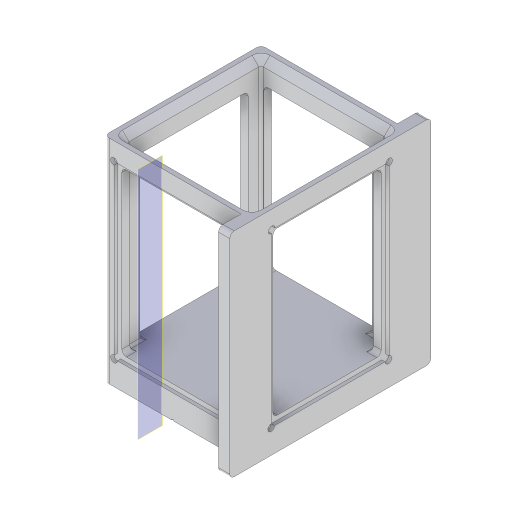
# Autodesk Inventor part: cuvette-w70mm-slide50x75mm-v1
Saved by Autodesk Inventor 2024 (Build 280153000, 153)
## iProperties
Created: 2025-09-30
Part Number: cuvette-w70mm-slide50x75mm-v1
Material: Generic
Document SubType Name: Modeling
Designer: N.Vladimirov
Density: 1 g/cm^3
Appearance: Default
Author: N.Vladimirov
Autodesk Inventor part; units mm, degrees
ref_plane "YZ Plane" through (0, 0, 0) normal (1, 0, 0) x (0, 1, 0)
ref_plane "XZ Plane" through (0, 0, 0) normal (0, 1, 0) x (-1, 0, 0)
ref_plane "XY Plane" through (0, 0, 0) normal (0, 0, 1) x (1, 0, 0)
sketch "Sketch1" plane through (0, 0, 0) normal (0, 0, 1) x (1, 0, 0)
  line L0 (30.5, -35) -> (-30.5, -35)
  line L1 (-30.5, -35) -> (-30.5, 35)
  line L2 (-30.5, 35) -> (30.5, 35)
  line L3 (30.5, 35) -> (30.5, -35)
  line L4 (30.5, -35) -> (-30.5, 35) construction
  line L5 (-30.5, -35) -> (30.5, 35) construction
  point P0 (0, 0)
  dimension "d0" = 61
  dimension "d1" = 70
  constraints: 12 end point, 2 midpoint, 2 parallel, 1 horizontal, 1 perpendicular
  measures "d0" distance of L1.end L2.end
  measures "d1" distance of L0.end L1.end
sketch "Sketch1 outline for Extrusion1" plane through (0, 0, 0) normal (0, 0, 1) x (1, 0, 0)
  line L0 (30.5, -35) -> (30.5, 35)
  line L1 (-30.5, -35) -> (30.5, -35)
  line L2 (-30.5, 35) -> (-30.5, -35)
  line L3 (30.5, 35) -> (-30.5, 35)
extrude "Extrusion1" add sketch "Sketch1 outline for Extrusion1" along normal blind 95.25
sketch "Sketch2" plane through (30.5, -35, 0) normal (1, 0, 0) x (0, 0, -1)
  line L0 (0, 0) -> (0, 70) projected
  line L1 (0, 70) -> (-95.25, 70) projected
  line L2 (-95.25, 0) -> (-95.25, 70) projected
  line L3 (0, 0) -> (-95.25, 0) projected
  line L4 (0, 70) -> (-95.25, 70) projected
  line L5 (-95.25, 70) -> (0, 70)
  line L6 (0, 70) -> (0, 80)
  line L7 (0, 80) -> (-95.25, 80)
  line L8 (-95.25, 80) -> (-95.25, 70)
  line L9 (-95.25, 70) -> (-95.25, 0) projected
  line L10 (-95.25, 0) -> (0, 0)
  line L11 (0, 0) -> (0, -10)
  line L12 (0, -10) -> (-95.25, -10)
  line L13 (-95.25, -10) -> (-95.25, 0)
  point P0 (0, 35)
  dimension "d4" = 10
  dimension "d5" = 10
  constraints: 16 end point, 4 parallel, 2 horizontal, 2 perpendicular, 1 point on line
  measures "d4" distance of L6.end L5.end
  measures "d5" distance of L10.end L11.end
sketch "Sketch2 outline for Extrusion2" plane through (30.5, -35, 0) normal (1, 0, 0) x (0, 0, -1)
  line L0 (-95.25, 80) -> (-95.25, 70)
  line L1 (0, 80) -> (-95.25, 80)
  line L2 (0, 70) -> (0, 80)
  line L3 (0, 0) -> (0, 70)
  line L4 (0, -10) -> (0, 0)
  line L5 (-95.25, -10) -> (0, -10)
  line L6 (-95.25, 0) -> (-95.25, -10)
  line L7 (-95.25, 70) -> (-95.25, 0)
extrude "Extrusion2" add sketch "Sketch2 outline for Extrusion2" along normal blind 5
sketch "Sketch12" plane through (35.5, -35, 0) normal (1, 0, 0) x (0, 0, -1)
  line L0 (-83.02098, 8.75) -> (-9.5, 8.75)
  line L1 (-8, 10.25) -> (-8, 59.75)
  line L2 (-9.5, 61.25) -> (-83.02098, 61.25)
  line L3 (-84.5, 60) -> (-84.5, 10.5)
  line L4 (-10, 57.25) -> (-10, 12.75)
  line L5 (-12, 10.75) -> (-80.5, 10.75)
  line L6 (-82.5, 12.75) -> (-82.5, 57.25)
  line L7 (-80.5, 59.25) -> (-12, 59.25)
  line L8 (0, -10) -> (0, 80)
  arc A0 (-10, 57.25) -> (-12, 59.25) centre (-12, 57.25) ccw
  arc A1 (-12, 10.75) -> (-10, 12.75) centre (-12, 12.75) ccw
  arc A2 (-82.5, 12.75) -> (-80.5, 10.75) centre (-80.5, 12.75) ccw
  arc A3 (-80.5, 59.25) -> (-82.5, 57.25) centre (-80.5, 57.25) ccw
  arc A4 (-8, 59.75) -> (-9.5, 61.25) centre (-8, 61.25) ccw
  arc A5 (-9.5, 8.75) -> (-8, 10.25) centre (-8, 8.75) ccw
  arc A6 (-83.02098, 61.25) -> (-84.5, 60) centre (-84.5, 61.5) ccw
  arc A7 (-84.5, 10.5) -> (-83.02098, 8.75) centre (-84.5, 9) ccw
  line L9 (0, 35) -> (-110.058309, 35)
  point P0 (0, -8)
  point P1 (0, 78)
  dimension "d57" = 2
  dimension "d58" = 8
  dimension "d59" = 2
  dimension "d60" = 3
  dimension "d61" = 3
  dimension "d62" = 3
  dimension "d63" = 3
  dimension "d119" = 2
  dimension "d120" = 76.5
  dimension "d121" = 52.5
  dimension "d122" = 2
  dimension "d123" = 2
  constraints: 18 end point, 16 point on circle, 8 centre point, 8 tangent, 4 parallel, 3 equal radius, 2 horizontal, 2 perpendicular, 1 other
  measures "d57" distance between parallel lines of L1 L4
  measures "d58" distance between parallel lines of L1 L8
  measures "d59" radius of A0
  measures "d60" diameter of A4
  measures "d61" diameter of A5
  measures "d62" diameter of A6
  measures "d63" diameter of A7
  measures "d119" distance between parallel lines of L3 L6
  measures "d120" distance between parallel lines of L3 L1
  measures "d121" distance between parallel lines of L0 L2
  measures "d122" distance between parallel lines of L7 L2
  measures "d123" distance between parallel lines of L5 L0
sketch "Sketch13" plane through (-30.5, -35, 0) normal (-1, 0, 0) x (0, 0, 1)
  line L0 (8, 10.25) -> (8, 59.75)
  line L1 (10, 57.25) -> (10, 12.75)
  line L2 (83.02098, 8.75) -> (9.5, 8.75)
  arc A0 (8, 10.25) -> (9.5, 8.75) centre (8, 8.75) ccw
  line L3 (12, 10.75) -> (80.5, 10.75)
  arc A1 (10, 12.75) -> (12, 10.75) centre (12, 12.75) ccw
  arc A2 (9.5, 61.25) -> (8, 59.75) centre (8, 61.25) ccw
  line L4 (9.5, 61.25) -> (83.02098, 61.25)
  line L5 (80.5, 59.25) -> (12, 59.25)
  line L6 (84.5, 60) -> (84.5, 10.5)
  line L7 (82.5, 12.75) -> (82.5, 57.25)
  arc A3 (84.5, 60) -> (83.02098, 61.25) centre (84.5, 61.5) ccw
  arc A4 (83.02098, 8.75) -> (84.5, 10.5) centre (84.5, 9) ccw
  arc A5 (80.5, 10.75) -> (82.5, 12.75) centre (80.5, 12.75) ccw
  arc A6 (82.5, 57.25) -> (80.5, 59.25) centre (80.5, 57.25) ccw
  arc A7 (12, 59.25) -> (10, 57.25) centre (12, 57.25) ccw
  point P0 (0, 35)
sketch "Sketch12 outline for Extrusion12" plane through (35.5, -35, 0) normal (1, 0, 0) x (0, 0, -1)
  arc A0 (-80.5, 59.25) -> (-82.5, 57.25) centre (-80.5, 57.25) ccw
  line L0 (-12, 59.25) -> (-80.5, 59.25)
  arc A1 (-10, 57.25) -> (-12, 59.25) centre (-12, 57.25) ccw
  line L1 (-10, 12.75) -> (-10, 57.25)
  arc A2 (-12, 10.75) -> (-10, 12.75) centre (-12, 12.75) ccw
  line L2 (-80.5, 10.75) -> (-12, 10.75)
  arc A3 (-82.5, 12.75) -> (-80.5, 10.75) centre (-80.5, 12.75) ccw
  line L3 (-82.5, 57.25) -> (-82.5, 12.75)
extrude "Extrusion12" cut sketch "Sketch12 outline for Extrusion12" against normal through all
ref_plane "LightSheet Plane1" through (-5.1, -35, 0) normal (-1, 0, 0) x (0, 0, 1)
sketch "Sketch15" plane through (-30.5, 35, 95.25) normal (0, 1, 0) x (1, 0, 0)
  line L0 (54.75, 10.75) -> (5.75, 10.75)
  line L1 (4.25, 12.25) -> (4.25, 85.75)
  line L2 (5.75, 87.25) -> (54.75, 87.25)
  line L3 (56.75, 85.835786) -> (56.75, 12.164214)
  line L4 (61, 95.25) -> (0, 95.25)
  line L5 (52.75, 85.25) -> (8.25, 85.25)
  line L6 (6.25, 83.25) -> (6.25, 14.75)
  line L7 (8.25, 12.75) -> (52.75, 12.75)
  line L8 (54.75, 14.75) -> (54.75, 83.25)
  arc A0 (8.25, 85.25) -> (6.25, 83.25) centre (8.25, 83.25) ccw
  arc A1 (54.75, 83.25) -> (52.75, 85.25) centre (52.75, 83.25) ccw
  arc A2 (52.75, 12.75) -> (54.75, 14.75) centre (52.75, 14.75) ccw
  arc A3 (6.25, 14.75) -> (8.25, 12.75) centre (8.25, 14.75) ccw
  arc A4 (5.75, 87.25) -> (4.25, 85.75) centre (4.25, 87.25) ccw
  arc A5 (56.75, 85.835786) -> (54.75, 87.25) centre (56.25, 87.25) ccw
  arc A6 (54.75, 10.75) -> (56.75, 12.164214) centre (56.25, 10.75) ccw
  arc A7 (4.25, 12.25) -> (5.75, 10.75) centre (4.25, 10.75) ccw
  line L9 (30.5, 95.25) -> (30.5, -2.042218)
  dimension "d84" = 8
  dimension "d85" = 2
  dimension "d86" = 2
  dimension "d87" = 3
  dimension "d88" = 3
  dimension "d89" = 3
  dimension "d90" = 3
  dimension "d124" = 52.5
  dimension "d125" = 76.5
  dimension "d126" = 2
  dimension "d127" = 2
  dimension "d128" = 2
  constraints: 18 end point, 16 point on circle, 8 centre point, 8 tangent, 4 parallel, 3 equal radius, 2 perpendicular, 1 horizontal, 1 vertical, 1 other
  measures "d84" distance between parallel lines of L2 L4
  measures "d85" distance between parallel lines of L2 L5
  measures "d86" radius of A0
  measures "d87" diameter of A4
  measures "d88" diameter of A5
  measures "d89" diameter of A6
  measures "d90" diameter of A7
  measures "d124" distance between parallel lines of L3 L1
  measures "d125" distance between parallel lines of L0 L2
  measures "d126" distance between parallel lines of L0 L7
  measures "d127" distance between parallel lines of L6 L1
  measures "d128" distance between parallel lines of L8 L3
sketch "Sketch15 outline for Extrusion16" plane through (-30.5, 35, 95.25) normal (0, 1, 0) x (1, 0, 0)
  line L0 (52.75, 85.25) -> (8.25, 85.25)
  arc A0 (54.75, 83.25) -> (52.75, 85.25) centre (52.75, 83.25) ccw
  line L1 (54.75, 14.75) -> (54.75, 83.25)
  arc A1 (52.75, 12.75) -> (54.75, 14.75) centre (52.75, 14.75) ccw
  line L2 (8.25, 12.75) -> (52.75, 12.75)
  arc A2 (6.25, 14.75) -> (8.25, 12.75) centre (8.25, 14.75) ccw
  line L3 (6.25, 83.25) -> (6.25, 14.75)
  arc A3 (8.25, 85.25) -> (6.25, 83.25) centre (8.25, 83.25) ccw
extrude "Extrusion16" cut sketch "Sketch15 outline for Extrusion16" against normal through all
sketch "Sketch16" plane through (-30.5, -35, 0) normal (0, -1, 0) x (1, 0, 0)
  line L0 (5.75, 8) -> (54.75, 8)
  arc A0 (4.25, 9.5) -> (5.75, 8) centre (4.25, 8) ccw
  line L1 (4.25, 83) -> (4.25, 9.5)
  arc A1 (54.75, 8) -> (56.75, 9.414214) centre (56.25, 8) ccw
  line L2 (56.75, 9.414214) -> (56.75, 83.085786)
  arc A2 (56.75, 83.085786) -> (54.75, 84.5) centre (56.25, 84.5) ccw
  line L3 (54.75, 84.5) -> (5.75, 84.5)
  arc A3 (5.75, 84.5) -> (4.25, 83) centre (4.25, 84.5) ccw
  point P0 (30.5, 0)
sketch "Sketch16 outline for Extrusion17" plane through (-30.5, -35, 0) normal (0, -1, 0) x (1, 0, 0)
  line L0 (5.75, 8) -> (54.75, 8)
  arc A0 (4.25, 9.5) -> (5.75, 8) centre (4.25, 8) ccw
  line L1 (4.25, 83) -> (4.25, 9.5)
  arc A1 (5.75, 84.5) -> (4.25, 83) centre (4.25, 84.5) ccw
  line L2 (54.75, 84.5) -> (5.75, 84.5)
  arc A2 (56.75, 83.085786) -> (54.75, 84.5) centre (56.25, 84.5) ccw
  line L3 (56.75, 9.414214) -> (56.75, 83.085786)
  arc A3 (54.75, 8) -> (56.75, 9.414214) centre (56.25, 8) ccw
extrude "Extrusion17" cut sketch "Sketch16 outline for Extrusion17" against normal blind 1.5
sketch "Sketch17" plane through (0, 0, 0) normal (0, 0, -1) x (-1, 0, 0)
  line L0 (25.5, 30) -> (-30.5, 30)
  line L1 (-30.5, 30) -> (-30.5, -30)
  line L2 (-30.5, -30) -> (25.5, -30)
  line L3 (25.5, -30) -> (25.5, 30)
  line L4 (-30.5, 35) -> (30.5, 35) projected
  line L5 (30.5, 35) -> (30.5, -35) projected
  line L6 (30.5, -35) -> (-30.5, -35) projected
  line L7 (-30.5, 35) -> (-30.5, 45) projected
  point P0 (0, 0)
  dimension "d95" = 5
  dimension "d96" = 5
  dimension "d97" = 5
  dimension "d98" = 0
  constraints: 8 end point, 2 parallel, 1 horizontal, 1 perpendicular
  measures "d95" distance between parallel lines of L0 L4
  measures "d96" distance between parallel lines of L3 L5
  measures "d97" distance between parallel lines of L6 L2
  measures "d98" distance between parallel lines of L7 L1
sketch "Sketch17 outline for Extrusion18" plane through (0, 0, 0) normal (0, 0, -1) x (-1, 0, 0)
  line L0 (25.5, 30) -> (-30.5, 30)
  line L1 (25.5, -30) -> (25.5, 30)
  line L2 (-30.5, -30) -> (25.5, -30)
  line L3 (-30.5, 30) -> (-30.5, -30)
extrude "Extrusion18" cut sketch "Sketch17 outline for Extrusion18" against normal up to surface (82.5 mm away)
fillet "Fillet2" radius 1 12 edges at (30.5, 26.125, 82.5) (26.375, 30, 82.5) (30.5, 30, 41.25) (30.5, -30, 41.25) (26.375, -30, 82.5) (30.5, -26.125, 82.5) (-25.5, -30, 41.25) (-25.5, 30, 41.25) (-25.5, -26.125, 82.5) (-25.5, 26.125, 82.5) (-23.875, 30, 82.5) (-23.875, -30, 82.5)
sketch "Sketch15 outline for Extrusion19" plane through (-30.5, 35, 95.25) normal (0, 1, 0) x (1, 0, 0)
  arc A0 (56.75, 85.835786) -> (54.75, 87.25) centre (56.25, 87.25) ccw
  line L0 (56.75, 12.164214) -> (56.75, 85.835786)
  arc A1 (54.75, 10.75) -> (56.75, 12.164214) centre (56.25, 10.75) ccw
  line L1 (5.75, 10.75) -> (54.75, 10.75)
  arc A2 (4.25, 12.25) -> (5.75, 10.75) centre (4.25, 10.75) ccw
  line L2 (4.25, 85.75) -> (4.25, 12.25)
  arc A3 (5.75, 87.25) -> (4.25, 85.75) centre (4.25, 87.25) ccw
  line L3 (54.75, 87.25) -> (5.75, 87.25)
extrude "Extrusion19" cut sketch "Sketch15 outline for Extrusion19" against normal blind 1.5
fillet "Fillet3" radius 2 4 edges at (33, 45, 0) (33, 45, 95.25) (33, -45, 0) (33, -45, 95.25)
sketch "Sketch12 outline for Extrusion20" plane through (35.5, -35, 0) normal (1, 0, 0) x (0, 0, -1)
  line L0 (-83.02098, 8.75) -> (-9.5, 8.75)
  arc A0 (-84.5, 10.5) -> (-83.02098, 8.75) centre (-84.5, 9) ccw
  line L1 (-84.5, 60) -> (-84.5, 10.5)
  arc A1 (-83.02098, 61.25) -> (-84.5, 60) centre (-84.5, 61.5) ccw
  line L2 (-9.5, 61.25) -> (-83.02098, 61.25)
  arc A2 (-8, 59.75) -> (-9.5, 61.25) centre (-8, 61.25) ccw
  line L3 (-8, 10.25) -> (-8, 59.75)
  arc A3 (-9.5, 8.75) -> (-8, 10.25) centre (-8, 8.75) ccw
extrude "Extrusion20" cut sketch "Sketch12 outline for Extrusion20" against normal blind 1.5
sketch "Sketch13 outline for Extrusion21" plane through (-30.5, -35, 0) normal (-1, 0, 0) x (0, 0, 1)
  arc A0 (83.02098, 8.75) -> (84.5, 10.5) centre (84.5, 9) ccw
  line L0 (9.5, 8.75) -> (83.02098, 8.75)
  arc A1 (8, 10.25) -> (9.5, 8.75) centre (8, 8.75) ccw
  line L1 (8, 59.75) -> (8, 10.25)
  arc A2 (9.5, 61.25) -> (8, 59.75) centre (8, 61.25) ccw
  line L2 (83.02098, 61.25) -> (9.5, 61.25)
  arc A3 (84.5, 60) -> (83.02098, 61.25) centre (84.5, 61.5) ccw
  line L3 (84.5, 10.5) -> (84.5, 60)
extrude "Extrusion21" cut sketch "Sketch13 outline for Extrusion21" against normal blind 1.5
sketch "Sketch18" plane through (0, 0, 95.25) normal (0, 0, 1) x (1, 0, 0)
  point P0 (0, 0)
  point P1 (0, 0)
  constraints: 1 coincident
hole "Hole2" at (0, 0, 95.25) direction (0, 0, -1) diameter 5.588 depth 10 tip angle 118 thread size "1/4-36 UNS" class "2B" standard "ANSI Unified Screw Threads"
sketch "Sketch19" plane through (-30.5, 35, 95.25) normal (0, 1, 0) x (1, 0, 0)
  circle A0 centre (30.5, 0) radius 0.5
  point P0 (30.5, 95.25)
  dimension "d116" = 1
  constraints: 1 centre point, 1 coincident
  measures "d116" diameter of A0
sketch "Sketch19 outline for Extrusion22" plane through (-30.5, 35, 95.25) normal (0, 1, 0) x (1, 0, 0)
  circle A0 centre (30.5, 0) radius 0.5
extrude "Extrusion22" cut sketch "Sketch19 outline for Extrusion22" against normal through all
chamfer "Chamfer1" distance 3 angle 45 8 edges at (-25.5, 0, 0) (-25.2071, -29.7071, 0) (2.5, -30, 0) (30.2071, -29.7071, 0) (30.5, 0, 0) (30.2071, 29.7071, 0) (2.5, 30, 0) (-25.2071, 29.7071, 0)
fillet "Fillet4" radius 2 2 edges at (-30.5, 35, 47.625) (-30.5, -35, 47.625)
body "Solid1"
